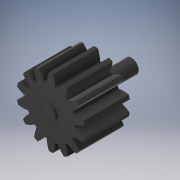
# Autodesk Inventor part: AC06
Saved by Autodesk Inventor 2017 SP1 (Build 210196100, 196)
## iProperties
Created: 2019-09-22
Part Number: AC06
Material: ABS Plastic
Document SubType Name: Modeling
Designer: Zach
Density: 1.06 g/cm^3
Appearance: Smooth - Black
Author: Zach
Autodesk Inventor part; units mm, degrees
ref_plane "YZ Plane" through (0, 0, 0) normal (1, 0, 0) x (0, 1, 0)
ref_plane "XZ Plane" through (0, 0, 0) normal (0, 1, 0) x (-1, 0, 0)
ref_plane "XY Plane" through (0, 0, 0) normal (0, 0, 1) x (1, 0, 0)
sketch "Sketch1" plane through (0, 0, 0) normal (0, 0, 1) x (1, 0, 0)
  arc A0 (5.9892, 8.4411) -> (6.9584, 12.5904) centre (-5.202, 13.243) ccw
  arc A1 (6.9584, 12.5904) -> (5.505, 13.2903) centre (0, 0) ccw
  arc A2 (5.505, 13.2903) -> (2.8652, 9.9455) centre (13.5971, 4.1898) ccw
  arc A3 (2.8652, 9.9455) -> (1.7337, 10.2038) centre (0, 0) ccw
  arc A4 (1.7337, 10.2038) -> (0.8066, 14.3627) centre (-10.4327, 9.6744) ccw
  arc A5 (0.8066, 14.3627) -> (-0.8066, 14.3627) centre (0, 0) ccw
  arc A6 (-0.8066, 14.3627) -> (-1.7337, 10.2038) centre (10.4327, 9.6744) ccw
  arc A7 (-1.7337, 10.2038) -> (-2.8652, 9.9455) centre (0, 0) ccw
  arc A8 (-2.8652, 9.9455) -> (-5.505, 13.2903) centre (-13.5971, 4.1898) ccw
  arc A9 (-5.505, 13.2903) -> (-6.9584, 12.5904) centre (0, 0) ccw
  arc A10 (-6.9584, 12.5904) -> (-5.9892, 8.4411) centre (5.202, 13.243) ccw
  arc A11 (-5.9892, 8.4411) -> (-6.8967, 7.7174) centre (0, 0) ccw
  arc A12 (-6.8967, 7.7174) -> (-10.7263, 9.5856) centre (-14.0685, -2.1247) ccw
  arc A13 (-10.7263, 9.5856) -> (-11.7321, 8.3244) centre (0, 0) ccw
  arc A14 (-11.7321, 8.3244) -> (-9.0586, 5.0065) centre (-1.0591, 14.1885) ccw
  arc A15 (-9.0586, 5.0065) -> (-9.5622, 3.9608) centre (0, 0) ccw
  arc A16 (-9.5622, 3.9608) -> (-13.8231, 3.9824) centre (-11.7534, -8.0184) ccw
  arc A17 (-13.8231, 3.9824) -> (-14.1821, 2.4096) centre (0, 0) ccw
  arc A18 (-14.1821, 2.4096) -> (-10.3337, 0.5803) centre (-7.1104, 12.3239) ccw
  arc A19 (-10.3337, 0.5803) -> (-10.3337, -0.5803) centre (0, 0) ccw
  arc A20 (-10.3337, -0.5803) -> (-14.1821, -2.4096) centre (-7.1104, -12.3239) ccw
  arc A21 (-14.1821, -2.4096) -> (-13.8231, -3.9824) centre (0, 0) ccw
  arc A22 (-13.8231, -3.9824) -> (-9.5622, -3.9608) centre (-11.7534, 8.0184) ccw
  arc A23 (-9.5622, -3.9608) -> (-9.0586, -5.0065) centre (0, 0) ccw
  arc A24 (-9.0586, -5.0065) -> (-11.7321, -8.3244) centre (-1.0591, -14.1885) ccw
  arc A25 (-11.7321, -8.3244) -> (-10.7263, -9.5856) centre (0, 0) ccw
  arc A26 (-10.7263, -9.5856) -> (-6.8967, -7.7174) centre (-14.0685, 2.1247) ccw
  arc A27 (-6.8967, -7.7174) -> (-5.9892, -8.4411) centre (0, 0) ccw
  arc A28 (-5.9892, -8.4411) -> (-6.9584, -12.5904) centre (5.202, -13.243) ccw
  arc A29 (-6.9584, -12.5904) -> (-5.505, -13.2903) centre (0, 0) ccw
  arc A30 (-5.505, -13.2903) -> (-2.8652, -9.9455) centre (-13.5971, -4.1898) ccw
  arc A31 (-2.8652, -9.9455) -> (-1.7337, -10.2038) centre (0, 0) ccw
  arc A32 (-1.7337, -10.2038) -> (-0.8066, -14.3627) centre (10.4327, -9.6744) ccw
  arc A33 (-0.8066, -14.3627) -> (0.8066, -14.3627) centre (0, 0) ccw
  arc A34 (0.8066, -14.3627) -> (1.7337, -10.2038) centre (-10.4327, -9.6744) ccw
  arc A35 (1.7337, -10.2038) -> (2.8652, -9.9455) centre (0, 0) ccw
  arc A36 (2.8652, -9.9455) -> (5.505, -13.2903) centre (13.5971, -4.1898) ccw
  arc A37 (5.505, -13.2903) -> (6.9584, -12.5904) centre (0, 0) ccw
  arc A38 (6.9584, -12.5904) -> (5.9892, -8.4411) centre (-5.202, -13.243) ccw
  arc A39 (5.9892, -8.4411) -> (6.8967, -7.7174) centre (0, 0) ccw
  arc A40 (6.8967, -7.7174) -> (10.7263, -9.5856) centre (14.0685, 2.1247) ccw
  arc A41 (10.7263, -9.5856) -> (11.7321, -8.3244) centre (0, 0) ccw
  arc A42 (11.7321, -8.3244) -> (9.0586, -5.0065) centre (1.0591, -14.1885) ccw
  arc A43 (9.0586, -5.0065) -> (9.5622, -3.9608) centre (0, 0) ccw
  arc A44 (9.5622, -3.9608) -> (13.8231, -3.9824) centre (11.7534, 8.0184) ccw
  arc A45 (13.8231, -3.9824) -> (14.1821, -2.4096) centre (0, 0) ccw
  arc A46 (14.1821, -2.4096) -> (10.3337, -0.5803) centre (7.1104, -12.3239) ccw
  arc A47 (10.3337, -0.5803) -> (10.3337, 0.5803) centre (0, 0) ccw
  arc A48 (10.3337, 0.5803) -> (14.1821, 2.4096) centre (7.1104, 12.3239) ccw
  arc A49 (14.1821, 2.4096) -> (13.8231, 3.9824) centre (0, 0) ccw
  arc A50 (13.8231, 3.9824) -> (9.5622, 3.9608) centre (11.7534, -8.0184) ccw
  arc A51 (9.5622, 3.9608) -> (9.0586, 5.0065) centre (0, 0) ccw
  arc A52 (9.0586, 5.0065) -> (11.7321, 8.3244) centre (1.0591, 14.1885) ccw
  arc A53 (11.7321, 8.3244) -> (10.7263, 9.5856) centre (0, 0) ccw
  arc A54 (10.7263, 9.5856) -> (6.8967, 7.7174) centre (14.0685, -2.1247) ccw
  arc A55 (6.8967, 7.7174) -> (5.9892, 8.4411) centre (0, 0) ccw
  constraints: 112 point on circle, 56 centre point
extrude "Extrusion1" add sketch "Sketch1" along normal blind 19
sketch "Sketch2" plane through (0, 0, 0) normal (0, 0, -1) x (-1, 0, 0)
  circle A0 centre (0, 0) radius 3
  dimension "d2" = 6
  constraints: 1 centre point, 1 coincident
  measures "d2" diameter of A0
extrude "Extrusion2" add sketch "Sketch2" along normal blind 15
sketch "Sketch3" plane through (0, 0, 19) normal (0, 0, 1) x (1, 0, 0)
  circle A0 centre (0, 0) radius 3
  dimension "d5" = 6
  constraints: 1 centre point, 1 coincident
  measures "d5" diameter of A0
extrude "Extrusion3" add sketch "Sketch3" along normal blind 1
body "Solid1"
